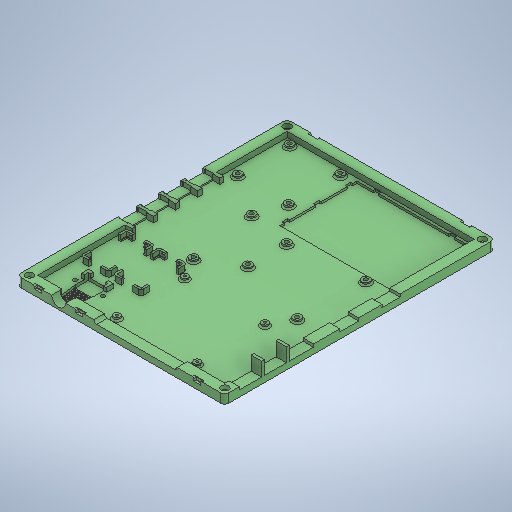
# Autodesk Inventor part: Electronic Base - Final
Saved by Autodesk Inventor 2025.2 (Build 292293000, 293)
## iProperties
Created: 2025-03-21
Part Number: Electronic Base - Final
Material: Generic
Document SubType Name: Modeling
Designer: mnguyen6
Density: 1 g/cm^3
Appearance: Default
Author: mnguyen6
Autodesk Inventor part; units mm, degrees
ref_plane "YZ Plane" through (0, 0, 0) normal (1, 0, 0) x (0, 1, 0)
ref_plane "XZ Plane" through (0, 0, 0) normal (0, 1, 0) x (-1, 0, 0)
ref_plane "XY Plane" through (0, 0, 0) normal (0, 0, 1) x (1, 0, 0)
sketch "Sketch1" plane through (0, 0, 0) normal (0, 1, 0) x (-1, 0, 0)
  line L0 (0, 0) -> (-135, 0)
  line L1 (-135, 0) -> (-135, 180)
  line L2 (-135, 180) -> (0, 180)
  line L3 (0, 180) -> (0, 0)
  line L4 (7.5, -7.5) -> (-142.5, -7.5)
  line L5 (-142.5, -7.5) -> (-142.5, 187.5)
  line L6 (-142.5, 187.5) -> (7.5, 187.5)
  line L7 (7.5, 187.5) -> (7.5, -7.5)
  line L8 (-31.4, 113) -> (-133, 113) construction
  line L9 (-133, 113) -> (-133, 59.66) construction
  line L10 (-133, 59.66) -> (-31.4, 59.66) construction
  line L11 (-31.4, 59.66) -> (-31.4, 113) construction
  circle A0 centre (-117.76, 110.46) radius 1.4
  circle A1 centre (-119.03, 62.2) radius 1.4
  circle A2 centre (-66.96, 95.22) radius 1.4
  circle A3 centre (-66.96, 67.28) radius 1.4
  circle A4 centre (-42.83, 110.46) radius 1.4
  circle A5 centre (-36.48, 62.2) radius 1.4
  circle A6 centre (-117.76, 110.46) radius 2.9
  circle A7 centre (-119.03, 62.2) radius 2.9
  circle A8 centre (-66.96, 67.28) radius 2.9
  circle A9 centre (-66.96, 95.22) radius 2.9
  circle A10 centre (-42.83, 110.46) radius 2.9
  circle A11 centre (-36.48, 62.2) radius 2.9
  line L12 (-134.5, 57.1943) -> (-52.82, 57.1943) construction
  line L13 (-52.82, 57.1943) -> (-52.82, 2.4443) construction
  line L14 (-52.82, 2.4443) -> (-134.5, 2.4443) construction
  line L15 (-134.5, 2.4443) -> (-134.5, 57.1943) construction
  line L16 (-52.32, 1.9443) -> (-52.32, 57.6943)
  line L17 (-52.32, 57.6943) -> (-135, 57.6943)
  line L18 (-135, 57.6943) -> (-135, 1.9443)
  line L19 (-135, 1.9443) -> (-52.32, 1.9443)
  line L20 (-52.32, 31.8193) -> (-50.82, 31.8193)
  line L21 (-50.82, 31.8193) -> (-50.82, 27.8193)
  line L22 (-50.82, 27.8193) -> (-52.32, 27.8193)
  line L23 (-52.32, 27.8193) -> (-52.32, 31.8193)
  line L24 (-52.32, 9.1193) -> (-50.82, 9.1193)
  line L25 (-50.82, 9.1193) -> (-50.82, 5.1193)
  line L26 (-50.82, 5.1193) -> (-52.32, 5.1193)
  line L27 (-52.32, 54.5193) -> (-50.82, 54.5193)
  line L28 (-50.82, 54.5193) -> (-50.82, 50.5193)
  line L29 (-50.82, 50.5193) -> (-52.32, 50.5193)
  line L30 (-118.6, 1.9443) -> (-122.6, 1.9443)
  line L31 (-122.6, 1.9443) -> (-122.6, 0.4443)
  line L32 (-122.6, 0.4443) -> (-118.6, 0.4443)
  line L33 (-118.6, 0.4443) -> (-118.6, 1.9443)
  line L34 (-68.07, 1.9443) -> (-64.07, 1.9443)
  line L35 (-64.07, 1.9443) -> (-64.07, 0.4443)
  line L36 (-64.07, 0.4443) -> (-68.07, 0.4443)
  line L37 (-68.07, 0.4443) -> (-68.07, 1.9443)
  line L38 (-48, 178) -> (-133, 178) construction
  line L39 (-133, 178) -> (-133, 122) construction
  line L40 (-133, 122) -> (-48, 122) construction
  line L41 (-48, 122) -> (-48, 178) construction
  circle A12 centre (-51.5, 174.5) radius 0.9
  circle A13 centre (-51.5, 125.5) radius 0.9
  circle A14 centre (-109.5, 174.5) radius 0.9
  circle A15 centre (-109.5, 125.5) radius 0.9
  circle A16 centre (-51.5, 174.5) radius 2.4
  circle A17 centre (-51.5, 125.5) radius 2.4
  circle A18 centre (-109.5, 174.5) radius 2.4
  circle A19 centre (-109.5, 125.5) radius 2.4
  line L42 (-4.5766, 150.6861) -> (-21.8766, 150.6861)
  line L43 (-21.8766, 150.6861) -> (-21.8766, 120.3861)
  line L44 (-21.8766, 120.3861) -> (-4.5766, 120.3861)
  line L45 (-4.5766, 120.3861) -> (-4.5766, 150.6861)
  line L46 (-3.2153, 44.9443) -> (-46.2153, 44.9443) construction
  line L47 (-46.2153, 44.9443) -> (-46.2153, 1.9443) construction
  line L48 (-46.2153, 1.9443) -> (-3.2153, 1.9443) construction
  line L49 (-3.2153, 1.9443) -> (-3.2153, 44.9443) construction
  line L50 (-27.8766, 150.6861) -> (-45.1766, 150.6861)
  line L51 (-45.1766, 150.6861) -> (-45.1766, 120.3861)
  line L52 (-45.1766, 120.3861) -> (-27.8766, 120.3861)
  line L53 (-27.8766, 120.3861) -> (-27.8766, 150.6861)
  circle A20 centre (-6.5353, 4.8153) radius 1.4
  circle A21 centre (-6.5353, 4.8153) radius 2.9
  circle A22 centre (-43.2723, 4.8153) radius 2.9
  circle A23 centre (-43.2723, 4.8153) radius 1.4
  circle A24 centre (-6.5353, 42.1883) radius 1.4
  circle A25 centre (-6.5353, 42.1883) radius 2.9
  circle A26 centre (-43.2723, 42.1883) radius 2.9
  circle A27 centre (-43.2723, 42.1883) radius 1.4
  line L54 (-22.5, 178.166) -> (-22.5, 163.2053) construction
  line L55 (-27.75, 181.5) -> (-29.5, 168.5)
  line L56 (-15.5, 168.5) -> (-17.25, 181.5)
  line L57 (-17.25, 181.5) -> (-27.75, 181.5)
  line L58 (-15.5, 168.5) -> (-15.5, 159)
  line L59 (-15.5, 159) -> (-29.5, 159)
  line L60 (-29.5, 159) -> (-29.5, 168.5)
  line L61 (-27.9654, 179.9) -> (-17.0346, 179.9)
  line L62 (-28.0731, 179.1) -> (-16.9269, 179.1)
  line L63 (-28.2346, 177.9) -> (-16.7654, 177.9)
  line L64 (-28.3423, 177.1) -> (-16.6577, 177.1)
  line L65 (-28.5038, 175.9) -> (-16.4962, 175.9)
  line L66 (-16.3885, 175.1) -> (-28.6115, 175.1)
  line L67 (-28.7731, 173.9) -> (-16.2269, 173.9)
  line L68 (-16.1192, 173.1) -> (-28.8808, 173.1)
  line L69 (-29.0423, 171.9) -> (-15.9577, 171.9)
  line L70 (-29.15, 171.1) -> (-15.85, 171.1)
  line L71 (-29.3115, 169.9) -> (-15.6885, 169.9)
  line L72 (-15.5808, 169.1) -> (-29.4192, 169.1)
  line L73 (-17.25, 159) -> (-27.75, 159)
  line L74 (-27.75, 159) -> (-27.75, 154.5)
  line L75 (-27.75, 154.5) -> (-17.25, 154.5)
  line L76 (-17.25, 154.5) -> (-17.25, 159)
  line L77 (-15.5, 162) -> (-13.5, 162)
  line L78 (-13.5, 162) -> (-13.5, 157)
  line L79 (-13.5, 157) -> (-17, 157)
  line L80 (-17, 157) -> (-17, 159)
  line L81 (-29.5, 162) -> (-31.5, 162)
  line L82 (-31.5, 162) -> (-31.5, 157)
  line L83 (-31.5, 157) -> (-28, 157)
  line L84 (-28, 157) -> (-28, 159)
  line L85 (-26.3766, 152.1861) -> (-46.6766, 152.1861)
  line L86 (-46.6766, 152.1861) -> (-46.6766, 118.8861)
  line L87 (-46.6766, 118.8861) -> (-26.3766, 118.8861)
  line L88 (-26.3766, 118.8861) -> (-26.3766, 152.1861)
  line L89 (-28.3766, 150.1861) -> (-44.6766, 150.1861)
  line L90 (-44.6766, 150.1861) -> (-44.6766, 120.8861)
  line L91 (-44.6766, 120.8861) -> (-28.3766, 120.8861)
  line L92 (-28.3766, 120.8861) -> (-28.3766, 150.1861)
  line L93 (-3.0766, 152.1861) -> (-23.3766, 152.1861)
  line L94 (-23.3766, 152.1861) -> (-23.3766, 118.8861)
  line L95 (-23.3766, 118.8861) -> (-3.0766, 118.8861)
  line L96 (-3.0766, 118.8861) -> (-3.0766, 152.1861)
  line L97 (-5.0766, 150.1861) -> (-21.3766, 150.1861)
  line L98 (-21.3766, 150.1861) -> (-21.3766, 120.8861)
  line L99 (-21.3766, 120.8861) -> (-5.0766, 120.8861)
  line L100 (-5.0766, 120.8861) -> (-5.0766, 150.1861)
  line L101 (-32.3766, 152.1861) -> (-32.3766, 150.1861)
  line L102 (-32.3766, 118.8861) -> (-32.3766, 120.8861)
  line L103 (-9.0766, 152.1861) -> (-9.0766, 150.1861)
  line L104 (-9.0766, 120.8861) -> (-9.0766, 118.8861)
  line L105 (-40.6766, 152.1861) -> (-40.6766, 150.1861)
  line L106 (-17.3766, 120.8861) -> (-17.3766, 118.8861)
  line L107 (-40.6766, 120.8861) -> (-40.6766, 118.8861)
  line L108 (-17.3766, 152.1861) -> (-17.3766, 150.1861)
  line L109 (-26.3766, 146.1861) -> (-28.3766, 146.1861)
  line L110 (-44.6766, 146.1861) -> (-46.6766, 146.1861)
  line L111 (-26.3766, 124.8861) -> (-28.3766, 124.8861)
  line L112 (-44.6766, 124.8861) -> (-46.6766, 124.8861)
  line L113 (-3.0766, 146.1861) -> (-5.0766, 146.1861)
  line L114 (-21.3766, 146.1861) -> (-23.3766, 146.1861)
  line L115 (-3.0766, 124.8861) -> (-5.0766, 124.8861)
  line L116 (-21.3766, 124.8861) -> (-23.3766, 124.8861)
  circle A28 centre (-12.5, 165.5) radius 1.5
  circle A29 centre (-32.5, 165.5) radius 1.5
  point P0 (-50.82, 29.8193)
  point P1 (-52.32, 29.8193)
  point P2 (-50.82, 7.1193)
  point P3 (-50.82, 52.5193)
  point P4 (-22.5, 154.5)
  point P5 (-22.5, 159)
  point P6 (-27.9519, 180)
  point P7 (-17.0481, 180)
  point P8 (-135, 1.9443)
  point P9 (-122.6, 1.9443)
  point P10 (-64.07, 1.9443)
  point P11 (-52.32, 5.1193)
  point P12 (-52.32, 27.8193)
  point P13 (-52.32, 54.5193)
  point P14 (-135, 57.6943)
  point P15 (-27.8766, 124.8861)
  point P16 (-32.3766, 120.3861)
  point P17 (-45.1766, 124.8861)
  point P18 (-40.6766, 120.3861)
  point P19 (-27.8766, 146.1861)
  point P20 (-32.3766, 150.6861)
  point P21 (-45.1766, 146.1861)
  point P22 (-40.6766, 150.6861)
  point P23 (-4.5766, 124.8861)
  point P24 (-9.0766, 120.3861)
  point P25 (-21.8766, 124.8861)
  point P26 (-17.3766, 120.3861)
  point P27 (-4.5766, 146.1861)
  point P28 (-9.0766, 150.6861)
  point P29 (-21.8766, 146.1861)
  point P30 (-17.3766, 150.6861)
  point P31 (-27.75, 159)
  point P32 (-28, 159)
  point P33 (-29.5, 162)
  dimension "d0" = 7.5
  dimension "d1" = 53.34
  dimension "d2" = 101.6
  dimension "d3" = 15.24
  dimension "d4" = 13.97
  dimension "d5" = 2.54
  dimension "d6" = 50.8
  dimension "d7" = 17.78
  dimension "d9" = 66.04
  dimension "d10" = 90.17
  dimension "d11" = 96.52
  dimension "d12" = 45.72
  dimension "d13" = 2.8
  dimension "d15" = 54.75
  dimension "d16" = 81.68
  dimension "d17" = 0.5
  dimension "d18" = 4
  dimension "d19" = 1.5
  dimension "d22" = 22.7
  dimension "d27" = 11.9
  dimension "d28" = 54.53
  dimension "d29" = 2
  dimension "d31" = 56
  dimension "d32" = 85
  dimension "d33" = 3.5
  dimension "d34" = 3.5
  dimension "d35" = 1.8
  dimension "d37" = 52.5
  dimension "d38" = 61.5
  dimension "d39" = 1.5
  dimension "d40" = 2
  dimension "d44" = 43
  dimension "d46" = 17.3
  dimension "d49" = 30.3
  dimension "d50" = 2.871
  dimension "d51" = 3.32
  dimension "d52" = 2.8
  dimension "d54" = 1.5
  dimension "d55" = 1.5
  dimension "d56" = 40.244
  dimension "d57" = 40.057
  dimension "d59" = 10.5
  dimension "d62" = 6
  dimension "d63" = 14
  dimension "d64" = 30
  dimension "d65" = 1.6
  dimension "d66" = 0.8
  dimension "d67" = 1.2
  dimension "d68" = 0.8
  dimension "d69" = 1.2
  dimension "d70" = 0.8
  dimension "d71" = 1.2
  dimension "d72" = 0.8
  dimension "d73" = 1.2
  dimension "d74" = 0.8
  dimension "d75" = 1.2
  dimension "d76" = 0.8
  dimension "d77" = 9.5
  dimension "d78" = 13
  dimension "d79" = 10.5
  dimension "d80" = 4.5
  dimension "d81" = 3
  dimension "d82" = 2
  dimension "d83" = 2
  constraints: 230 end point, 41 parallel, 38 point on line, 30 centre point, 27 perpendicular, 23 horizontal, 22 equal radius, 13 coincident, 13 collinear, 10 vertical, 8 equal length, 8 horizontal alignment, 6 symmetric about line, 6 vertical alignment, 4 midpoint, 65 other
  measures "d0" distance between parallel lines of L3 L7
  measures "d1" distance of L8.end L9.end
  measures "d2" distance of L9.end L10.end
  measures "d3" distance from line of L9 A0.centre
  measures "d4" distance from line of L9 A1.centre
  measures "d5" distance from line of L8 A0.centre
  measures "d6" distance from line of A1.centre L8
  measures "d7" distance from line of A2.centre L8
  measures "d9" distance from line of L9 A2.centre
  measures "d10" horizontal distance of L9.end A4.centre
  measures "d11" horizontal distance of L9.end A5.centre
  measures "d12" vertical distance of L8.end A3.centre
  measures "d13" diameter of A0
  measures "d15" distance of L14.end L12.start
  measures "d16" distance of L13.end L14.end
  measures "d17" distance between parallel lines of L13 L16
  measures "d18" distance of L20.end L21.end
  measures "d19" distance of L21.end L22.end
  measures "d22" distance of L20.start L24.start
  measures "d27" distance between parallel lines of L15 L31
  measures "d28" distance of L31.end L36.end
  measures "d29" distance between parallel lines of L1 L9
  measures "d31" distance of L38.end L39.end
  measures "d32" distance of L38.start L38.end
  measures "d33" distance from line of L38 A12.centre
  measures "d34" distance from line of L41 A12.centre
  measures "d35" diameter of A12
  measures "d37" vertical distance of L38.start A13.centre
  measures "d38" distance from line of L41 A14.centre
  measures "d39" radial gap between concentric circles of A12 A16
  measures "d40" distance between parallel lines of L2 L38
  measures "d44" distance of L46.end L47.end
  measures "d46" distance of L50.start L50.end
  measures "d49" distance of L50.end L51.end
  measures "d50" distance from line of L48 A20.centre
  measures "d51" horizontal distance of L48.end A20.centre
  measures "d52" diameter of A20
  measures "d54" radial gap between concentric circles of A21 A20
  measures "d55" radial gap between concentric circles of A6 A0
  measures "d56" distance from line of A24.centre L48
  measures "d57" horizontal distance of A22.centre L48.end
  measures "d59" distance of L57.start L57.end
  measures "d62" distance between parallel lines of L6 L57
  measures "d63" distance of L58.end L59.end
  measures "d64" distance between parallel lines of L7 L54
  measures "d65" distance between parallel lines of L57 L61
  measures "d66" distance between parallel lines of L61 L62
  measures "d67" distance between parallel lines of L63 L62
  measures "d68" distance between parallel lines of L64 L63
  measures "d69" distance between parallel lines of L64 L65
  measures "d70" distance between parallel lines of L65 L66
  measures "d71" distance between parallel lines of L66 L67
  measures "d72" distance between parallel lines of L67 L68
  measures "d73" distance between parallel lines of L68 L69
  measures "d74" distance between parallel lines of L69 L70
  measures "d75" distance between parallel lines of L70 L71
  measures "d76" distance between parallel lines of L71 L72
  measures "d77" distance of L58.end L58.start
  measures "d78" vertical distance of L57.start L58.start
  measures "d79" distance of L74.end L75.end
  measures "d80" distance of L73.end L74.end
  measures "d81" distance of L58.end L77.start
  measures "d82" distance of L77.start L77.end
  measures "d83" distance of L79.end L80.end
extrude "Base" add sketch "Sketch1" against normal blind 2.5 contours L0 L1 L19 L31 L32 L33 L37 L36 L35 L16 L26 L25 L24 L22 L21 L20 L29 L28 L27 L17 L2 L55 L60 L81 L82 L83 L84 L59 L74 L75 L76 L80 L79 L78 L77 L58 L56 L3 | L1 L17 L16 L19 | L56 L61 L55 L2 | L2 L55 L57 L56 | L19 L33 L32 L31 | L56 L62 L55 L61 | L56 L63 L55 L62 | L27 L28 L29 L16 | L19 L35 L36 L37 | L56 L64 L55 L63 | L56 L65 L55 L64 | L20 L21 L22 L16 | L56 L66 L55 L65 | L16 L24 L25 L26 | L56 L67 L55 L66 | L56 L68 L55 L67 | L56 L69 L55 L68 | L56 L70 L55 L69 | L56 L71 L55 L70 | L56 L72 L55 L71 | L56 L58 L59 L60 L55 L72 | L77 L78 L79 L80 L59 L58 | L60 L59 L84 L83 L82 L81 | L76 L75 L74 L59 | L4 L5 L6 L7 | A0 | A1 | A2 | A3 | A4 | A5 | A6 | A7 | A8 | A9 | A10 | A11 | A12 | A13 | A14 | A15 | A16 | A17 | A18 | A19 | L45 L113 L100 L97 L103 L42 | L42 L103 L93 L96 L113 L45 | L103 L97 L108 L42 | L42 L108 L93 L103 | L113 L96 L115 L45 | L45 L115 L100 L113 | L108 L97 L98 L114 L43 L42 | L42 L43 L114 L94 L93 L108 | L97 L100 L99 L98 | L115 L96 L95 L104 L44 L45 | L45 L44 L104 L99 L100 L115 | L114 L98 L116 L43 | L43 L116 L94 L114 | L104 L95 L106 L44 | L44 L106 L99 L104 | L116 L98 L99 L106 L44 L43 | L43 L44 L106 L95 L94 L116 | L53 L109 L92 L89 L101 L50 | L50 L101 L85 L88 L109 L53 | L101 L89 L105 L50 | L50 L105 L85 L101 | L109 L88 L111 L53 | L53 L111 L92 L109 | L105 L89 L90 L110 L51 L50 | L50 L51 L110 L86 L85 L105 | L89 L92 L91 L90 | L111 L88 L87 L102 L52 L53 | L53 L52 L102 L91 L92 L111 | L110 L90 L112 L51 | L51 L112 L86 L110 | L102 L87 L107 L52 | L52 L107 L91 L102 | L112 L90 L91 L107 L52 L51 | L51 L52 L107 L87 L86 L112 | A20 | A21 | A22 | A23 | A24 | A25 | A26 | A27 | A28 | A29
extrude "Wall" add sketch "Sketch1" along normal blind 4 contours L4 L5 L6 L7
extrude "Breadboard slot" cut sketch "Sketch1" against normal blind 1.5 contours L1 L17 L16 L19 | L19 L33 L32 L31 | L27 L28 L29 L16 | L19 L35 L36 L37 | L20 L21 L22 L16 | L16 L24 L25 L26
extrude "Electronic mounting holes" add sketch "Sketch1" along normal blind 2 contours A6 | A7 | A8 | A9 | A10 | A11 | A16 | A17 | A18 | A19 | A21 | A22 | A25 | A26
chamfer "Chamfer1" distance 1 angle 45 14 edges at (53.9, 0, 174.5) (111.9, 0, 174.5) (53.9, 0, 125.5) (111.9, 0, 125.5) (120.66, 0, 110.46) (69.86, 0, 95.22) (45.73, 0, 110.46) (69.86, 0, 67.28) (39.38, 0, 62.2) (46.1723, 0, 42.1883) (121.93, 0, 62.2) (9.4353, 0, 42.1883) (9.4353, 0, 4.8153) (46.1723, 0, 4.8153)
extrude "Deeper mounting holes" cut sketch "Sketch1" against normal blind 1 contours A0 | A1 | A2 | A3 | A4 | A5 | A12 | A13 | A14 | A15 | A20 | A23 | A24 | A27
extrude "Extrusion14" cut sketch "Sketch1" against normal through all contours A28 | A29
extrude "MT3608 base" add sketch "Sketch1" along normal blind 1 contours L45 L113 L100 L97 L103 L42 | L108 L97 L98 L114 L43 L42 | L45 L44 L104 L99 L100 L115 | L116 L98 L99 L106 L44 L43 | L53 L109 L92 L89 L101 L50 | L105 L89 L90 L110 L51 L50 | L53 L52 L102 L91 L92 L111 | L112 L90 L91 L107 L52 L51
extrude "MT3608 wall" add sketch "Sketch1" along normal blind 4 contours L42 L103 L93 L96 L113 L45 | L42 L43 L114 L94 L93 L108 | L115 L96 L95 L104 L44 L45 | L43 L44 L106 L95 L94 L116 | L50 L101 L85 L88 L109 L53 | L50 L51 L110 L86 L85 L105 | L111 L88 L87 L102 L52 L53 | L51 L52 L107 L87 L86 L112
sketch "Sketch2" plane through (32.3766, 0, 150.1861) normal (1, 0, 0) x (0, 0, -1)
  line L0 (-0.5, 1) -> (-0.5, 4) projected
  line L1 (-0.5, 4) -> (0.25, 3.25)
  line L2 (0.25, 3.25) -> (-0.5, 2.5)
  line L3 (0.25, 3.25) -> (-0.5, 3.25) construction
  point P0 (150.1861, 0)
  dimension "d108" = 1.5
  dimension "d109" = 45
  constraints: 6 end point, 1 midpoint, 1 perpendicular, 1 point on line, 1 other
  measures "d108" distance of L0.start L2.end
  measures "d109" angle of L0 L2
extrude "MT3608 snap" add sketch "Sketch2" against normal blind 2
ref_plane "Work Plane1" through (32.3766, 0, 135.5361) normal (0, 0, -1) x (-1, 0, 0)
ref_plane "Work Plane2" through (36.5266, 0, 152.1861) normal (-1, 0, 0) x (0, 0, 1)
fillet "Fillet1" radius 0.3 1 edges at (31.3766, 3.25, 149.9361)
mirror "Mirror1" about plane through (32.3766, 0, 135.5361) normal (0, 0, -1) of "MT3608 snap", "Fillet1"
mirror "Mirror2" about plane through (36.5266, 0, 152.1861) normal (-1, 0, 0) of "MT3608 snap", "Mirror1", "Fillet1"
ref_plane "Work Plane3" through (24.8766, 0, 146.1861) normal (1, 0, 0) x (0, 0, -1)
mirror "Mirror3" about plane through (24.8766, 0, 146.1861) normal (1, 0, 0) of "MT3608 snap", "Fillet1", "Mirror1", "Mirror2"
fillet "Fillet2" radius 2 8 edges at (26.3766, 2, 152.1861) (26.3766, 2, 118.8861) (3.0766, 2, 152.1861) (3.0766, 2, 118.8861) (46.6766, 2, 152.1861) (46.6766, 2, 118.8861) (23.3766, 2, 152.1861) (23.3766, 2, 118.8861)
extrude "Extrusion9" cut sketch "Sketch1" against normal blind 2 contours L56 L61 L55 L2 | L2 L55 L57 L56 | L56 L62 L55 L61 | L56 L63 L55 L62 | L56 L64 L55 L63 | L56 L65 L55 L64 | L56 L66 L55 L65 | L56 L67 L55 L66 | L56 L68 L55 L67 | L56 L69 L55 L68 | L56 L70 L55 L69 | L56 L71 L55 L70 | L56 L72 L55 L71 | L56 L58 L59 L60 L55 L72
extrude "Extrusion10" add sketch "Sketch1" along normal blind 0.5 from surface at -2 contours L56 L61 L55 L2 | L56 L62 L55 L61 | L56 L64 L55 L63 | L56 L66 L55 L65 | L56 L68 L55 L67 | L56 L70 L55 L69 | L56 L72 L55 L71
extrude "Extrusion11" add sketch "Sketch1" along normal blind 3 contours L77 L78 L79 L80 L59 L58 | L60 L59 L84 L83 L82 L81
sketch "Sketch4" plane through (0, 4, 0) normal (0, 1, 0) x (1, 0, 0)
  line L0 (142.5, -187.5) -> (142.5, 7.5) projected
  line L1 (135, 0) -> (135, -180) projected
  line L2 (48, -178) -> (133, -178) construction
  line L3 (135, -177) -> (142.5, -177)
  line L4 (142.5, -177) -> (142.5, -161)
  line L5 (142.5, -161) -> (135, -161)
  line L6 (135, -161) -> (135, -177)
  line L7 (135, -159) -> (142.5, -159)
  line L8 (142.5, -159) -> (142.5, -143)
  line L9 (142.5, -143) -> (135, -143)
  line L10 (135, -143) -> (135, -159)
  line L11 (135, -141) -> (142.5, -141)
  line L12 (142.5, -141) -> (142.5, -123.5)
  line L13 (142.5, -123.5) -> (135, -123.5)
  line L14 (135, -123.5) -> (135, -141)
  line L15 (31.4, -113) -> (133, -113) construction
  line L16 (135, -104.5) -> (142.5, -104.5)
  line L17 (142.5, -104.5) -> (142.5, -90.86)
  line L18 (142.5, -90.86) -> (135, -90.86)
  line L19 (135, -90.86) -> (135, -104.5)
  line L20 (135, -74) -> (142.5, -74)
  line L21 (142.5, -74) -> (142.5, -61)
  line L22 (142.5, -61) -> (135, -61)
  line L23 (135, -61) -> (135, -74)
  line L24 (-7.5, -187.5) -> (142.5, -187.5) projected
  line L25 (135, -180) -> (27.9519, -180) projected
  line L26 (48, -187.5) -> (108, -187.5)
  line L27 (108, -187.5) -> (108, -180)
  line L28 (108, -180) -> (48, -180)
  line L29 (48, -180) -> (48, -187.5)
  line L30 (133, -178) -> (133, -122) construction
  point P0 (135, -61)
  point P1 (142.5, -104.5)
  point P2 (142.5, -177)
  point P3 (108, -187.5)
  dimension "d125" = 1
  dimension "d127" = 19
  dimension "d129" = 37
  dimension "d131" = 8.5
  dimension "d132" = 13.64
  dimension "d133" = 39
  dimension "d134" = 13
  dimension "d137" = 25
  dimension "d138" = 85
  dimension "d176" = 17
  dimension "d177" = 35
  dimension "d178" = 54.5
  constraints: 48 end point, 12 parallel, 12 point on line, 6 horizontal, 6 perpendicular
  measures "d125" distance from line of L3.end L2
  measures "d127" vertical distance of L2.end L7.end
  measures "d129" vertical distance of L2.end L11.end
  measures "d131" vertical distance of L15.end L16.end
  measures "d132" distance of L16.end L17.end
  measures "d133" vertical distance of L20.end L15.end
  measures "d134" distance of L20.end L21.end
  measures "d137" horizontal distance of L2.end L26.end
  measures "d138" distance from line of L30 L26.start
  measures "d176" distance between parallel lines of L5 L2
  measures "d177" distance between parallel lines of L2 L9
  measures "d178" distance from line of L2.end L13
extrude "Board Ports" cut sketch "Sketch4" against normal blind 2 contours L3 L1 L5 L0 | L24 L29 L25 L27 | L7 L1 L9 L0 | L11 L1 L13 L0 | L16 L1 L18 L0 | L20 L1 L22 L0
fillet "Fillet6" radius 2 2 edges at (48, 2, 183.75) (108, 2, 183.75)
extrude "Extrusion22" add sketch "Sketch4" along normal blind 8 contours L5 L1 L7 L0 | L9 L1 L11 L0
sketch "Sketch5" plane through (27.75, 4, 181.5) normal (0, 0, -1) x (-1, 0, 0)
  line L0 (0, 0) -> (10.5, 0) projected
  line L1 (0, -6) -> (10.5, -6) projected
  circle A0 centre (5.25, 0) radius 5
  point P0 (27.75, -4)
  point P1 (5.25, -5)
  point P2 (5.25, -5)
  dimension "d139" = 10
  constraints: 1 centre point, 1 midpoint
  measures "d139" diameter of A0
extrude "DC jack opening" cut sketch "Sketch5" against normal through all
fillet "Fillet3" radius 3 4 edges at (-7.5, 0.75, 187.5) (-7.5, 0.75, -7.5) (142.5, 0.75, 187.5) (142.5, 0.75, -7.5)
ref_plane "Work Plane4" through (122.5, 4, 123.5) normal (1, 0, 0) x (0, 0, -1)
ref_plane "Work Plane5" through (37.5, 4, 123.5) normal (1, 0, 0) x (0, 0, -1)
ref_plane "Work Plane6" through (12.5, 4, 123.5) normal (1, 0, 0) x (0, 0, -1)
ref_plane "Work Plane7" through (7.5, 4, 123.5) normal (1, 0, 0) x (0, 0, -1)
sketch "Sketch6" plane through (142.5, 4, 123.5) normal (1, 0, 0) x (0, 0, -1)
  line L0 (128, -6.5) -> (-61, -6.5) projected
  line L1 (-64, 0) -> (-56.5, 0) projected
  line L2 (-64, 0) -> (-62.5, 0)
  line L3 (-62.5, 0) -> (-62.5, -2.5)
  line L4 (-62.5, -2.5) -> (-64, -2.5)
  line L5 (-64, -2.5) -> (-64, 0)
  line L6 (-62.5, -2.5) -> (-61.5, -1.5)
  line L7 (-61.5, -1.5) -> (-62.5, -0.5)
  line L8 (-61.5, -1.5) -> (-62.5, -1.5) construction
  line L9 (33.5, 7.7447) -> (33.5, -39.6927) construction
  line L10 (131, 0) -> (129.5, 0)
  line L11 (129.5, 0) -> (129.5, -2.5)
  line L12 (129.5, -2.5) -> (131, -2.5)
  line L13 (131, -2.5) -> (131, 0)
  line L14 (129.5, -2.5) -> (128.5, -1.5)
  line L15 (128.5, -1.5) -> (129.5, -0.5)
  line L16 (128.5, -1.5) -> (129.5, -1.5) construction
  point P0 (123.5, -4)
  point P1 (33.5, -6.5)
  point P2 (-62.5, 0)
  dimension "d148" = 1.5
  dimension "d149" = 2.5
  dimension "d150" = 1
  dimension "d151" = 45
  constraints: 30 end point, 7 symmetric about line, 5 point on line, 2 parallel, 2 perpendicular, 1 horizontal, 1 midpoint, 1 vertical, 1 other
  measures "d148" distance of L1.start L2.end
  measures "d149" distance of L4.end L1.start
  measures "d150" distance of L6.end L8.end
  measures "d151" angle of L3 L6
extrude "Snap fit point 1" cut sketch "Sketch6" along normal mid plane 5 from surface at -20 contours L1 L3 L4 L5 | L7 L6 L3
extrude "Snap fit point 2" cut sketch "Sketch6" along normal mid plane 5 from surface at -105 contours L1 L3 L4 L5 | L7 L6 L3
extrude "Snap fit point 3" cut sketch "Sketch6" along normal mid plane 5 from surface at -135 contours L1 L3 L4 L5 | L7 L6 L3
extrude "Snap fit point 4" cut sketch "Sketch6" along normal mid plane 5 from surface at -130 contours L13 L12 L11 L10 | L11 L14 L15
extrude "Snap fit point 5" cut sketch "Sketch6" along normal mid plane 5 from surface at -20 contours L13 L12 L11 L10 | L11 L14 L15
fillet "Fillet4" radius 1 5 edges at (122.5, 2.5, 185) (37.5, 2.5, 185) (7.5, 2.5, 185) (122.5, 2.5, -5) (12.5, 2.5, -5)
fillet "Fillet5" radius 1 10 edges at (10, 4, -6.75) (15, 4, -6.75) (120, 4, -6.75) (125, 4, -6.75) (125, 4, 186.75) (120, 4, 186.75) (40, 4, 186.75) (35, 4, 186.75) (10, 4, 186.75) (5, 4, 186.75)
sketch "Sketch12" plane through (0, -2.5, 0) normal (0, -1, 0) x (1, 0, 0)
  line L0 (139.5, 187.5) -> (-4.5, 187.5) projected
  line L1 (-7.5, 184.5) -> (-7.5, -4.5) projected
  line L2 (-0.1, 181.3257) -> (-3, 179.6514)
  line L3 (-3, 179.6514) -> (-5.9, 181.3257)
  line L4 (-5.9, 181.3257) -> (-5.9, 184.6743)
  line L5 (-5.9, 184.6743) -> (-3, 186.3486)
  line L6 (-3, 186.3486) -> (-0.1, 184.6743)
  line L7 (-0.1, 184.6743) -> (-0.1, 181.3257)
  circle A0 centre (-3, 183) radius 2.75
  circle A1 centre (-3, 183) radius 1.6
  point P0 (0, 0)
  dimension "d189" = 5.8
  dimension "d190" = 4.5
  dimension "d191" = 4.5
  dimension "d192" = 5.5
  dimension "d195" = 3.2
  constraints: 12 end point, 2 centre point, 2 coincident, 1 vertical, 13 other
  measures "d189" distance between parallel lines of L2 L5
  measures "d190" distance from line of L0 point (-3, 183)
  measures "d191" distance from line of L1 point (-3, 183)
  measures "d192" diameter of A0
  measures "d195" diameter of A1
extrude "Extrusion24" cut sketch "Sketch12" against normal blind 1 contours L2 L3 L4 L5 L6 L7 | A0 | A1
extrude "Extrusion25" cut sketch "Sketch12" against normal through all contours A1
extrude "Base mounting hole" cut sketch "Sketch12" along normal blind 3 from surface at -6.5 contours A0
ref_plane "Work Plane8" through (48, 2, 90) normal (0, 0, 1) x (1, 0, 0)
ref_plane "Work Plane9" through (67.5, -2.5, -4.5) normal (-1, 0, 0) x (0, 0, 1)
mirror "Mirror4" about plane through (67.5, -2.5, -4.5) normal (-1, 0, 0) of "Extrusion25", "Extrusion24", "Base mounting hole"
mirror "Mirror5" about plane through (48, 2, 90) normal (0, 0, 1) of "Base mounting hole", "Extrusion25", "Extrusion24", "Mirror4"
sketch "Sketch13" plane through (0, 0, 0) normal (0, 1, 0) x (1, 0, 0)
  line L0 (24.94, -154.5283) -> (2.3635, -154.5283)
  line L1 (2.3635, -154.5283) -> (2.3635, -117.6302)
  line L2 (2.3635, -117.6302) -> (24.94, -117.6302)
  line L3 (24.94, -117.6302) -> (24.94, -154.5283)
  line L4 (24.94, -154.5283) -> (2.3635, -117.6302) construction
  line L5 (2.3635, -154.5283) -> (24.94, -117.6302) construction
  point P0 (13.6517, -136.0793)
  constraints: 12 end point, 2 midpoint, 2 parallel, 1 horizontal, 1 perpendicular
extrude "MT3608 snap fit test" [suppressed]
ref_plane "Work Plane10" through (0, 4, 0) normal (0, 1, 0) x (1, 0, 0)
sketch "Sketch14" plane through (0, 4, 0) normal (0, 1, 0) x (1, 0, 0)
  line L0 (-6.2, -115) -> (0, -115)
  line L1 (0, -115) -> (0, -101)
  line L2 (0, -101) -> (-6.2, -101)
  line L3 (-6.2, -101) -> (-6.2, -115)
  line L4 (-7.5, 4.5) -> (-7.5, -184.5) projected
  line L5 (-7.5, -114.45) -> (0, -114.45)
  line L6 (0, -114.45) -> (0, -101.55)
  line L7 (0, -101.55) -> (-7.5, -101.55)
  line L8 (-7.5, -101.55) -> (-7.5, -114.45)
  line L9 (-8.1019, -108) -> (2.4668, -108) construction
  line L10 (0, -180) -> (0, 0) projected
  line L11 (-3.75, -105.2483) -> (-3.75, -121.6196) construction
  point P0 (-3.1, -101)
  point P1 (-3.75, -101.55)
  point P2 (-6.2, -101.55)
  point P3 (-7.5, -101.55)
  point P4 (-6.2, -114.45)
  point P5 (0, -114.45)
  point P6 (0, -101.55)
  dimension "d203" = 6.2
  dimension "d204" = 14
  dimension "d205" = 12.9
  dimension "d213" = 115
  dimension "d224" = 1.3
  constraints: 20 end point, 4 parallel, 3 horizontal, 3 point on line, 2 midpoint, 2 perpendicular, 1 vertical, 2 other
  measures "d203" distance of L0.start L0.end
  measures "d204" distance between parallel lines of L2 L0
  measures "d205" distance between parallel lines of L7 L5
  measures "d213" distance from line of L10.end L0
  measures "d224" distance between parallel lines of L4 L3
extrude "DC Motor JST-PH Slot" cut sketch "Sketch14" against normal blind 3
sketch "Sketch16" plane through (0, 4, 0) normal (0, 1, 0) x (1, 0, 0)
  line L0 (0, 0) -> (0, -180) projected
  line L1 (0, -117) -> (5, -117)
  line L2 (5, -117) -> (5, -99)
  line L3 (5, -99) -> (0, -99)
  line L4 (0, -99) -> (0, -117)
  line L5 (-8.1019, -108) -> (2.4668, -108) construction
  line L6 (-7.5, -114.45) -> (0, -114.45) projected
  line L7 (0, -101.55) -> (-7.5, -101.55) projected
  line L8 (0, -114.45) -> (5, -114.45)
  line L9 (0, -101.55) -> (5, -101.55)
  line L10 (-6.2, -115) -> (0, -115) projected
  line L11 (0, -115) -> (0, -101) projected
  line L12 (0, -101) -> (-6.2, -101) projected
  point P0 (0, -99)
  point P1 (0, -114.45)
  point P2 (0, -115)
  point P3 (0, -101)
  point P4 (0, -101.55)
  dimension "d225" = 9
  dimension "d226" = 5
  constraints: 12 end point, 3 parallel, 3 point on line, 2 perpendicular, 1 horizontal, 1 other
  measures "d225" distance between parallel lines of L3 L5
  measures "d226" distance of L1.start L1.end
extrude "JST-PH reinforce" add sketch "Sketch16" against normal up to surface (4 mm away) contours L3 L2 L9 L0 | L8 L2 L1 L0
pattern_linear "Rectangular Pattern2" count 4 spacing 16 along (0, 0, -1) of "DC Motor JST-PH Slot", "JST-PH reinforce"
pattern_linear "Rectangular Pattern1" count 4 spacing 16 along (0, 0, -1) of "DC Motor JST-PH Slot"
sketch "Sketch17" plane through (0, 4, 0) normal (0, 1, 0) x (1, 0, 0)
  line L0 (-8.1181, -119.1634) -> (7.5083, -119.1634)
  line L1 (7.5083, -119.1634) -> (7.5083, -95.6299)
  line L2 (7.5083, -95.6299) -> (-8.1181, -95.6299)
  line L3 (-8.1181, -95.6299) -> (-8.1181, -119.1634)
  point P0 (0, 0)
  constraints: 8 end point, 2 parallel, 1 horizontal, 1 perpendicular
extrude "JST-PH Connector Test" [suppressed]
equation "\"d1\" = MEGA_width"
equation "\"d2\" = MEGA_length"
equation "\"d3\" = MEGA_hole1_y"
equation "\"d4\" = MEGA_hole2_y"
equation "\"d5\" = MEGA_hole1_x"
equation "\"d6\" = MEGA_hole2_x"
equation "\"d7\" = MEGA_hole3_x"
equation "\"d9\" = MEGA_hole3_y"
equation "\"d10\" = MEGA_hole5_y"
equation "\"d11\" = MEGA_hole6_y"
equation "\"d12\" = MEGA_hole4_x"
equation "\"d29\" = base_border"
equation "\"d31\" = Pi_width"
equation "\"d32\" = Pi_length"
equation "\"d33\" = Pi_hole1_x"
equation "\"d34\" = Pi_hole1_y"
equation "\"d37\" = Pi_hole2_x"
equation "\"d38\" = Pi_hole3_y"
equation "\"d40\" = base_border"
equation "\"d44\" = L298N_width"
equation "\"MEGA_width\" = 53.34"
equation "\"MEGA_length\" = 101.6"
equation "\"MEGA_hole1_y\" = 15.24"
equation "\"MEGA_hole1_x\" = 2.54"
equation "\"MEGA_hole2_x\" = 50.8"
equation "\"MEGA_hole2_y\" = 13.97"
equation "\"MEGA_hole3_x\" = 17.78"
equation "\"MEGA_hole3_y\" = 66.04"
equation "\"MEGA_hole4_x\" = 45.72"
equation "\"MEGA_hole5_y\" = 90.17"
equation "\"MEGA_hole6_y\" = 96.52"
equation "\"Pi_width\" = 56"
equation "\"Pi_length\" = 85"
equation "\"Pi_hole1_x\" = 3.5"
equation "\"Pi_hole1_y\" = 3.5"
equation "\"Pi_hole2_x\" = 52.5"
equation "\"Pi_hole3_y\" = 61.5"
equation "\"base_border\" = 2"
equation "\"MT3608_width\" = 17"
equation "\"L298N_width\" = 43"
equation "\"d48\" = 17"
equation "\"mount_hole_wall\" = 1.5"
body "Solid1"
